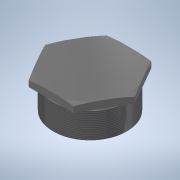
# Autodesk Inventor part: Korek sześciokątny BSP 4'' L=55
Saved by Autodesk Inventor 2020 (Build 240168000, 168)
## iProperties
RuleStatus: InUse
Created: 2022-03-21
Part Number: Korek sześciokątny BSP 4'' L=55
Material: 304
Description: Korek sześciokątny BSP 4'' L=55
Document SubType Name: Modelowanie
Designer: Radosław
Density: 8 g/cm^3
Sheet Metal Rule: 1,5
Sheet Metal Width: 0,000 mm
Sheet Metal Length: 0,000 mm
Sheet Metal Area: 0,000 mm^2
Appearance: Częściowo polerowany(1)
Author: Radosław
Autodesk Inventor part; units mm, degrees
ref_plane "YZ Plane" through (0, 0, 0) normal (1, 0, 0) x (0, 1, 0)
ref_plane "XZ Plane" through (0, 0, 0) normal (0, 1, 0) x (-1, 0, 0)
ref_plane "XY Plane" through (0, 0, 0) normal (0, 0, 1) x (1, 0, 0)
sketch "Szkic7" plane through (0, 0, 0) normal (0, 0, 1) x (1, 0, 0)
  circle A0 centre (0, 0) radius 56.515
  dimension "d35" = 113.03
  constraints: 1 centre point, 1 coincident
  measures "d35" diameter of A0
extrude "Wyciągnięcie proste2" add sketch "Szkic7" along normal mid plane 40.5625
chamfer "Faza2" distance 1 angle 45 1 edges at (-56.515, 0, 20.2812)
sketch "Szkic9" plane through (0, 0, 20.2812) normal (0, 0, 1) x (1, 0, 0)
  circle A0 centre (0, 0) radius 55.515 projected
extrude "Wyciągnięcie proste3" add sketch "Szkic9" along normal blind 3.4375
sketch "Szkic10" plane through (0, 0, 23.7188) normal (0, 0, 1) x (1, 0, 0)
  line L0 (-34.3523, 59.5) -> (34.3523, 59.5)
  line L1 (34.3523, 59.5) -> (68.7047, 0)
  line L2 (68.7047, 0) -> (34.3523, -59.5)
  line L3 (34.3523, -59.5) -> (-34.3523, -59.5)
  line L4 (-34.3523, -59.5) -> (-68.7047, 0)
  line L5 (-68.7047, 0) -> (-34.3523, 59.5)
  line L6 (0, 79.121) -> (0, -79.121) construction
  line L7 (-79.121, 0) -> (79.121, 0) construction
  point P0 (0, 0)
  point P1 (0, 0)
  point P2 (0, 59.5)
  dimension "d44" = 119
  constraints: 12 end point, 2 point on line, 1 coincident, 1 midpoint, 13 other
  measures "d44" distance between parallel lines of L4 L1
extrude "Wyciągnięcie proste4" add sketch "Szkic10" along normal blind 11
sketch "Szkic12" plane through (0, 0, 0) normal (0, 1, 0) x (-1, 0, 0)
  line L0 (0, -2.1463) -> (0, 12.8775) construction
  line L1 (-34.3523, 23.7188) -> (-34.3523, 34.7188) construction
  line L2 (-68.7047, 34.7188) -> (-34.3523, 34.7188) construction
  line L3 (-68.7047, 23.7188) -> (-68.7047, 34.7188) projected
  line L4 (-68.7047, 32.593) -> (-60.7713, 34.7188)
  line L5 (-68.7047, 34.7188) -> (-34.3523, 34.7188) projected
  line L6 (-68.7047, 23.7188) -> (-34.3523, 23.7188) projected
  point P0 (0, 0)
  dimension "d50" = 15
  dimension "d51" = 7.9333
  constraints: 2 end point, 2 point on line
  measures "d50" angle of L2 L4
  measures "d51" distance from line of L3 L4.end
revolve "Obrót2" cut sketch "Szkic12" angle 360 about axis through (0, 0, -10) along (0, 0, 1)
thread "Gwint3" size "G113.03x2.309" designation "G 4" class "A" standard "ISO Pipe Threads" full length
chamfer "Faza3" distance 1 angle 45 1 edges at (-56.515, 0, -20.2812)
equation "\"d35\" = OD"
equation "\"d36\" = 0.7375 * L"
equation "\"d42\" = 0.0625 * L"
equation "\"d44\" = SW"
equation "\"d45\" = 0.2 * L"
equation "\"d51\" = 0.0666667 * SW"
equation "\"SzerokośćGięciaPodcięcia\" = Grubość"
equation "\"RozmiarPodcięciaNarożnika\" = 4 * Grubość"
equation "\"PromieńPrzejścia\" = PromieńGięcia"
equation "\"Rozmiar_promienia_Jacobiego\" = PromieńGięcia"
equation "\"Wielk_odstępu\" = Grubość"
equation "\"d2\" = PromieńGięcia"
equation "\"d23\" = PromieńGięcia"
equation "\"OD\" = 113.03"
equation "\"SW\" = 119"
equation "\"L\" = 55"
equation "\"Grubość\" = 1.5"
equation "\"PromieńGięcia\" = 3"
